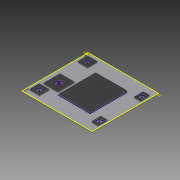
# Autodesk Inventor part: Back_part
Saved by Autodesk Inventor 2015 SP2 (Build 190223200, 223)
## iProperties
Created: 2016-11-11
Part Number: Back_part
Material: Generic
Document SubType Name: Modeling
Designer: Yann Cesbron
Density: 1 g/cm^3
Appearance: Default
Mass: 3708.65 g
Surface Area: 8125 cm^2
Volume: 3708.65 cm^3
Material: Perspex Black 9961 -10 mm
Author: Yann Cesbron
Autodesk Inventor part; units mm, degrees
ref_plane "YZ Plane" through (0, 0, 0) normal (1, 0, 0) x (0, 1, 0)
ref_plane "XZ Plane" through (0, 0, 0) normal (0, 1, 0) x (-1, 0, 0)
ref_plane "XY Plane" through (0, 0, 0) normal (0, 0, 1) x (1, 0, 0)
ref_plane "Work Plane1" through (0, 0, 0) normal (0, 0, 1) x (1, 0, 0)
sketch "Sketch1" plane through (0, 0, 0) normal (0, 0, 1) x (1, 0, 0)
  point P0 (0, 0)
ref_plane "Work Plane2" through (0, 0, 0) normal (0, 0, 1) x (1, 0, 0)
sketch "Sketch2" plane through (0, 0, 0) normal (0, 0, 1) x (1, 0, 0)
  line L0 (0, 10) -> (620, 10)
  line L1 (620, 10) -> (620, -575)
  line L2 (620, -575) -> (0, -575)
  line L3 (0, -575) -> (0, 10)
  point P0 (0, 0)
  dimension "d0" = 620
  dimension "d1" = 585
  dimension "d2" = 620
  dimension "d254" = 10
  constraints: 8 end point, 2 parallel, 1 horizontal, 1 perpendicular
  measures "d0" distance of L1.end L2.end
  measures "d1" distance between parallel lines of L0 L2
  measures "d2" distance from line of point (0, 0) L1
  measures "d254" distance from line of point (0, 0) L0
extrude "Extrusion1" add sketch "Sketch2" along normal blind 10
sketch "Excitation_port" plane through (0, 0, 10) normal (0, 0, 1) x (1, 0, 0)
  circle A0 centre (110, -357) radius 13
  line L0 (0, 10) -> (0, -575) projected
  line L1 (0, -575) -> (620, -575) projected
  circle A1 centre (110, -357) radius 30
  point P0 (0, 0)
  dimension "d6" = 26
  dimension "d7" = 110
  dimension "d8" = 218
  dimension "d9" = 60
  constraints: 2 centre point, 1 concentric
  measures "d6" diameter of A0
  measures "d7" distance from line of L0 A0.centre
  measures "d8" distance from line of L1 A0.centre
  measures "d9" diameter of A1
sketch "Air_duct_shapes_back" plane through (0, 0, 10) normal (0, 0, 1) x (1, 0, 0)
  circle A0 centre (75, -70) radius 23.5
  line L0 (0, 10) -> (0, -575) projected
  line L1 (620, 10) -> (0, 10) projected
  circle A1 centre (580, -470) radius 23.5
  circle A2 centre (580, -95) radius 23.5
  circle A3 centre (75, -495) radius 23.5
  line L2 (0, -575) -> (620, -575) projected
  line L3 (620, -575) -> (620, 10) projected
  point P0 (0, 0)
  dimension "d10" = 47
  dimension "d11" = 75
  dimension "d12" = 80
  dimension "d13" = 47
  dimension "d14" = 47
  dimension "d15" = 47
  dimension "d16" = 80
  dimension "d17" = 75
  dimension "d18" = 105
  dimension "d19" = 105
  dimension "d20" = 40
  dimension "d21" = 40
  constraints: 4 centre point
  measures "d10" diameter of A0
  measures "d11" distance from line of L0 A0.centre
  measures "d12" distance from line of L1 A0.centre
  measures "d13" diameter of A1
  measures "d14" diameter of A2
  measures "d15" diameter of A3
  measures "d16" distance from line of L2 A3.centre
  measures "d17" distance from line of L0 A3.centre
  measures "d18" distance from line of L2 A1.centre
  measures "d19" distance from line of L1 A2.centre
  measures "d20" distance from line of L3 A2.centre
  measures "d21" distance from line of L3 A1.centre
sketch "Flanges_back" plane through (0, 0, 10) normal (0, 0, 1) x (1, 0, 0)
  line L0 (620, -575) -> (620, 10) projected
  circle A0 centre (580, -95) radius 23.75
  line L1 (605, -52.5) -> (555, -52.5)
  line L2 (550, -57.5) -> (550, -132.5)
  line L3 (555, -137.5) -> (605, -137.5)
  line L4 (610, -132.5) -> (610, -57.5)
  line L5 (610, -52.5) -> (550, -137.5) construction
  line L6 (550, -52.5) -> (610, -137.5) construction
  line L7 (620, 10) -> (0, 10) projected
  circle A1 centre (580, -470) radius 23.75
  line L8 (0, -575) -> (620, -575) projected
  line L9 (555, -512.5) -> (605, -512.5)
  line L10 (610, -507.5) -> (610, -432.5)
  line L11 (605, -427.5) -> (555, -427.5)
  line L12 (550, -432.5) -> (550, -507.5)
  line L13 (550, -512.5) -> (610, -427.5) construction
  line L14 (610, -512.5) -> (550, -427.5) construction
  circle A2 centre (75, -70) radius 23.75
  line L15 (0, 10) -> (0, -575) projected
  line L16 (35, -115) -> (115, -115)
  line L17 (120, -110) -> (120, -30)
  line L18 (115, -25) -> (35, -25)
  line L19 (30, -30) -> (30, -110)
  line L20 (30, -115) -> (120, -25) construction
  line L21 (120, -115) -> (30, -25) construction
  circle A3 centre (75, -495) radius 23.75
  line L22 (35, -540) -> (115, -540)
  line L23 (120, -535) -> (120, -455)
  line L24 (115, -450) -> (35, -450)
  line L25 (30, -455) -> (30, -535)
  line L26 (30, -540) -> (120, -450) construction
  line L27 (120, -540) -> (30, -450) construction
  circle A4 centre (110, -357) radius 30
  line L28 (50, -432) -> (170, -432)
  line L29 (175, -427) -> (175, -287)
  line L30 (170, -282) -> (50, -282)
  line L31 (45, -287) -> (45, -427)
  line L32 (45, -432) -> (175, -282) construction
  line L33 (175, -432) -> (45, -282) construction
  circle A5 centre (602.5, -60) radius 2.25
  circle A6 centre (557.5, -60) radius 2.25
  circle A7 centre (557.5, -130) radius 2.25
  circle A8 centre (602.5, -130) radius 2.25
  circle A9 centre (602.5, -505) radius 2.25
  circle A10 centre (602.5, -435) radius 2.25
  circle A11 centre (557.5, -435) radius 2.25
  circle A12 centre (557.5, -505) radius 2.25
  circle A13 centre (75, -32.5) radius 2.25
  circle A14 centre (112.5, -70) radius 2.25
  circle A15 centre (75, -107.5) radius 2.25
  circle A16 centre (37.5, -70) radius 2.25
  circle A17 centre (112.5, -495) radius 2.25
  circle A18 centre (75, -532.5) radius 2.25
  circle A19 centre (75, -457.5) radius 2.25
  circle A20 centre (37.5, -495) radius 2.25
  circle A21 centre (167.5, -317) radius 2.25
  circle A22 centre (167.5, -397) radius 2.25
  circle A23 centre (110, -424.5) radius 2.25
  circle A24 centre (110, -289.5) radius 2.25
  circle A25 centre (52.5, -317) radius 2.25
  circle A26 centre (52.5, -397) radius 2.25
  arc A27 (115, -115) -> (120, -110) centre (115, -110) ccw
  arc A28 (120, -30) -> (115, -25) centre (115, -30) ccw
  arc A29 (35, -25) -> (30, -30) centre (35, -30) ccw
  arc A30 (30, -110) -> (35, -115) centre (35, -110) ccw
  arc A31 (115, -540) -> (120, -535) centre (115, -535) ccw
  arc A32 (120, -455) -> (115, -450) centre (115, -455) ccw
  arc A33 (35, -450) -> (30, -455) centre (35, -455) ccw
  arc A34 (30, -535) -> (35, -540) centre (35, -535) ccw
  arc A35 (175, -287) -> (170, -282) centre (170, -287) ccw
  arc A36 (50, -282) -> (45, -287) centre (50, -287) ccw
  arc A37 (45, -427) -> (50, -432) centre (50, -427) ccw
  arc A38 (170, -432) -> (175, -427) centre (170, -427) ccw
  arc A39 (550, -507.5) -> (555, -512.5) centre (555, -507.5) ccw
  arc A40 (605, -512.5) -> (610, -507.5) centre (605, -507.5) ccw
  arc A41 (610, -432.5) -> (605, -427.5) centre (605, -432.5) ccw
  arc A42 (555, -427.5) -> (550, -432.5) centre (555, -432.5) ccw
  arc A43 (555, -52.5) -> (550, -57.5) centre (555, -57.5) ccw
  arc A44 (610, -57.5) -> (605, -52.5) centre (605, -57.5) ccw
  arc A45 (605, -137.5) -> (610, -132.5) centre (605, -132.5) ccw
  arc A46 (550, -132.5) -> (555, -137.5) centre (555, -132.5) ccw
  point P0 (0, 0)
  point P1 (580, -95)
  point P2 (580, -470)
  point P3 (75, -495)
  point P4 (110, -357)
  dimension "d69" = 47.5
  dimension "d70" = 105
  dimension "d71" = 60
  dimension "d72" = 85
  dimension "d75" = 47.5
  dimension "d76" = 40
  dimension "d77" = 105
  dimension "d78" = 60
  dimension "d79" = 85
  dimension "d80" = 40
  dimension "d81" = 47.5
  dimension "d82" = 80
  dimension "d83" = 75
  dimension "d84" = 90
  dimension "d86" = 47.5
  dimension "d87" = 80
  dimension "d88" = 75
  dimension "d91" = 60
  dimension "d92" = 130
  dimension "d93" = 150
  dimension "d94" = 110
  dimension "d95" = 218
  dimension "d109" = 4.5
  dimension "d110" = 7.5
  dimension "d111" = 7.5
  dimension "d112" = 4.5
  dimension "d113" = 7.5
  dimension "d114" = 7.5
  dimension "d115" = 4.5
  dimension "d116" = 7.5
  dimension "d117" = 7.5
  dimension "d118" = 4.5
  dimension "d119" = 7.5
  dimension "d120" = 7.5
  dimension "d135" = 4.5
  dimension "d136" = 4.5
  dimension "d137" = 4.5
  dimension "d138" = 4.5
  dimension "d139" = 7.5
  dimension "d140" = 7.5
  dimension "d141" = 7.5
  dimension "d142" = 7.5
  dimension "d143" = 7.5
  dimension "d144" = 7.5
  dimension "d145" = 7.5
  dimension "d146" = 7.5
  dimension "d170" = 4.5
  dimension "d171" = 4.5
  dimension "d172" = 4.5
  dimension "d173" = 4.5
  dimension "d174" = 7.5
  dimension "d175" = 7.5
  dimension "d176" = 7.5
  dimension "d177" = 7.5
  dimension "d178" = 45
  dimension "d179" = 45
  dimension "d180" = 45
  dimension "d181" = 45
  dimension "d194" = 4.5
  dimension "d195" = 4.5
  dimension "d196" = 4.5
  dimension "d197" = 4.5
  dimension "d198" = 7.5
  dimension "d199" = 7.5
  constraints: 60 end point, 47 centre point, 40 point on circle, 40 point on line, 40 tangent, 16 midpoint, 15 equal radius, 10 parallel, 7 perpendicular, 5 coincident, 5 horizontal
  measures "d69" diameter of A0
  measures "d70" distance from line of L7 A0.centre
  measures "d71" distance of L5.end L6.end
  measures "d72" distance between parallel lines of L3 L1
  measures "d75" diameter of A1
  measures "d76" distance from line of L0 A1.centre
  measures "d77" distance from line of L8 A1.centre
  measures "d78" distance of L14.end L13.end
  measures "d79" distance of L13.end L14.start
  measures "d80" distance from line of L0 point (580, -95)
  measures "d81" diameter of A2
  measures "d82" distance from line of L7 A2.centre
  measures "d83" distance from line of L15 A2.centre
  measures "d84" distance of L21.end L20.end
  measures "d86" diameter of A3
  measures "d87" distance from line of L8 A3.centre
  measures "d88" distance from line of L15 A3.centre
  measures "d91" diameter of A4
  measures "d92" distance of L33.end L32.end
  measures "d93" distance of L32.end L33.start
  measures "d94" distance from line of L15 A4.centre
  measures "d95" distance from line of L8 A4.centre
  measures "d109" diameter of A5
  measures "d110" distance from line of L4 A5.centre
  measures "d111" distance from line of L1 A5.centre
  measures "d112" diameter of A6
  measures "d113" distance from line of L2 A6.centre
  measures "d114" distance from line of L1 A6.centre
  measures "d115" diameter of A7
  measures "d116" distance from line of L3 A7.centre
  measures "d117" distance from line of L2 A7.centre
  measures "d118" diameter of A8
  measures "d119" distance from line of L3 A8.centre
  measures "d120" distance from line of L4 A8.centre
  measures "d135" diameter of A9
  measures "d136" diameter of A10
  measures "d137" diameter of A11
  measures "d138" diameter of A12
  measures "d139" distance from line of A9.centre L9
  measures "d140" distance from line of L10 A9.centre
  measures "d141" distance from line of L10 A10.centre
  measures "d142" distance from line of L11 A10.centre
  measures "d143" distance from line of L12 A11.centre
  measures "d144" distance from line of L11 A11.centre
  measures "d145" distance from line of L9 A12.centre
  measures "d146" distance from line of L12 A12.centre
  measures "d170" diameter of A13
  measures "d171" diameter of A14
  measures "d172" diameter of A15
  measures "d173" diameter of A16
  measures "d174" distance from line of L17 A14.centre
  measures "d175" distance from line of L16 A15.centre
  measures "d176" distance from line of L18 A13.centre
  measures "d177" distance from line of L19 A16.centre
  measures "d178" distance from line of A14.centre L18
  measures "d179" distance from line of L17 A15.centre
  measures "d180" distance from line of L16 A16.centre
  measures "d181" distance from line of L19 A13.centre
  measures "d194" diameter of A17
  measures "d195" diameter of A18
  measures "d196" diameter of A19
  measures "d197" diameter of A20
  measures "d198" distance from line of L23 A17.centre
  measures "d199" distance from line of L22 A18.centre
sketch "Cut_out_back" plane through (0, 0, 10) normal (0, 0, 1) x (1, 0, 0)
  line L0 (620, 10) -> (0, 10) projected
  line L1 (0, 10) -> (0, -575) projected
  line L2 (557.5, -67.5) -> (602.5, -67.5)
  line L3 (607.5, -72.5) -> (607.5, -117.5)
  line L4 (602.5, -122.5) -> (557.5, -122.5)
  line L5 (552.5, -117.5) -> (552.5, -72.5)
  line L6 (552.5, -67.5) -> (607.5, -122.5) construction
  line L7 (607.5, -67.5) -> (552.5, -122.5) construction
  line L8 (557.5, -442.5) -> (602.5, -442.5)
  line L9 (607.5, -447.5) -> (607.5, -492.5)
  line L10 (602.5, -497.5) -> (557.5, -497.5)
  line L11 (552.5, -492.5) -> (552.5, -447.5)
  line L12 (552.5, -442.5) -> (607.5, -497.5) construction
  line L13 (607.5, -442.5) -> (552.5, -497.5) construction
  line L14 (0, -575) -> (620, -575) projected
  line L15 (620, -575) -> (620, 10) projected
  arc A0 (552.5, -117.5) -> (557.5, -122.5) centre (557.5, -117.5) ccw
  arc A1 (557.5, -67.5) -> (552.5, -72.5) centre (557.5, -72.5) ccw
  arc A2 (607.5, -72.5) -> (602.5, -67.5) centre (602.5, -72.5) ccw
  arc A3 (602.5, -122.5) -> (607.5, -117.5) centre (602.5, -117.5) ccw
  arc A4 (557.5, -442.5) -> (552.5, -447.5) centre (557.5, -447.5) ccw
  arc A5 (607.5, -447.5) -> (602.5, -442.5) centre (602.5, -447.5) ccw
  arc A6 (602.5, -497.5) -> (607.5, -492.5) centre (602.5, -492.5) ccw
  arc A7 (552.5, -492.5) -> (557.5, -497.5) centre (557.5, -492.5) ccw
  line L16 (65, -417) -> (155, -417)
  line L17 (160, -412) -> (160, -302)
  line L18 (155, -297) -> (65, -297)
  line L19 (60, -302) -> (60, -412)
  line L20 (60, -417) -> (160, -297) construction
  line L21 (160, -417) -> (60, -297) construction
  arc A8 (65, -297) -> (60, -302) centre (65, -302) ccw
  arc A9 (160, -302) -> (155, -297) centre (155, -302) ccw
  arc A10 (155, -417) -> (160, -412) centre (155, -412) ccw
  arc A11 (60, -412) -> (65, -417) centre (65, -412) ccw
  line L22 (100, -40) -> (50, -40)
  line L23 (45, -45) -> (45, -95)
  line L24 (50, -100) -> (100, -100)
  line L25 (105, -95) -> (105, -45)
  line L26 (105, -40) -> (45, -100) construction
  line L27 (45, -40) -> (105, -100) construction
  arc A12 (100, -100) -> (105, -95) centre (100, -95) ccw
  arc A13 (105, -45) -> (100, -40) centre (100, -45) ccw
  arc A14 (50, -40) -> (45, -45) centre (50, -45) ccw
  arc A15 (45, -95) -> (50, -100) centre (50, -95) ccw
  line L28 (100, -465) -> (50, -465)
  line L29 (45, -470) -> (45, -520)
  line L30 (50, -525) -> (100, -525)
  line L31 (105, -520) -> (105, -470)
  line L32 (105, -465) -> (45, -525) construction
  line L33 (45, -465) -> (105, -525) construction
  arc A16 (100, -525) -> (105, -520) centre (100, -520) ccw
  arc A17 (105, -470) -> (100, -465) centre (100, -470) ccw
  arc A18 (50, -465) -> (45, -470) centre (50, -470) ccw
  arc A19 (45, -520) -> (50, -525) centre (50, -520) ccw
  circle A20 centre (602.5, -130) radius 1.65
  circle A21 centre (602.5, -60) radius 1.65
  circle A22 centre (557.5, -60) radius 1.65
  circle A23 centre (557.5, -130) radius 1.65
  circle A24 centre (602.5, -505) radius 1.65
  circle A25 centre (557.5, -505) radius 1.65
  circle A26 centre (557.5, -435) radius 1.65
  circle A27 centre (602.5, -435) radius 1.65
  circle A28 centre (112.5, -70) radius 1.65
  circle A29 centre (75, -32.5) radius 1.65
  circle A30 centre (37.5, -70) radius 1.65
  circle A31 centre (75, -107.5) radius 1.65
  circle A32 centre (112.5, -495) radius 1.65
  circle A33 centre (37.5, -495) radius 1.65
  circle A34 centre (75, -532.5) radius 1.65
  circle A35 centre (75, -457.5) radius 1.65
  circle A36 centre (167.5, -317) radius 1.65
  circle A37 centre (167.5, -397) radius 1.65
  circle A38 centre (110, -424.5) radius 1.65
  circle A39 centre (52.5, -397) radius 1.65
  circle A40 centre (52.5, -317) radius 1.65
  circle A41 centre (110, -289.5) radius 1.65
  line L34 (0, 10) -> (20, 10)
  line L35 (20, 10) -> (20, -35)
  line L36 (20, -35) -> (0, -35)
  line L37 (0, -35) -> (0, 10)
  line L38 (0, -575) -> (20, -575)
  line L39 (20, -575) -> (20, -530)
  line L40 (20, -530) -> (0, -530)
  line L41 (0, -530) -> (0, -575)
  circle A42 centre (35, 5) radius 2.25
  circle A43 centre (170, 5) radius 2.25
  circle A44 centre (305, 5) radius 2.25
  circle A45 centre (440, 5) radius 2.25
  circle A46 centre (575, 5) radius 2.25
  circle A47 centre (35, -570) radius 2.25
  circle A48 centre (170, -570) radius 2.25
  circle A49 centre (305, -570) radius 2.25
  circle A50 centre (440, -570) radius 2.25
  circle A51 centre (575, -570) radius 2.25
  circle A52 centre (615, -30) radius 2.25
  circle A53 centre (615, -195) radius 2.25
  circle A54 centre (615, -370) radius 2.25
  circle A55 centre (615, -535) radius 2.25
  line L42 (220, -432.5) -> (450, -432.5)
  line L43 (460, -422.5) -> (460, -142.5)
  line L44 (450, -132.5) -> (220, -132.5)
  line L45 (210, -142.5) -> (210, -422.5)
  line L46 (210, -432.5) -> (460, -132.5) construction
  line L47 (460, -432.5) -> (210, -132.5) construction
  arc A56 (450, -432.5) -> (460, -422.5) centre (450, -422.5) ccw
  arc A57 (460, -142.5) -> (450, -132.5) centre (450, -142.5) ccw
  arc A58 (220, -132.5) -> (210, -142.5) centre (220, -142.5) ccw
  arc A59 (210, -422.5) -> (220, -432.5) centre (220, -422.5) ccw
  point P0 (0, 0)
  point P1 (580, -95)
  point P2 (580, -470)
  point P3 (110, -357)
  point P4 (75, -70)
  point P5 (75, -495)
  point P6 (335, -282.5)
  point P7 (467.5, -147.5)
  point P8 (467.5, -417.5)
  point P9 (445, -125)
  point P10 (445, -440)
  point P11 (225, -440)
  point P12 (202.5, -417.5)
  point P13 (202.5, -147.5)
  point P14 (225, -125)
  point P15 (335, -125)
  point P16 (467.5, -282.5)
  point P17 (335, -440)
  point P18 (202.5, -282.5)
  dimension "d26" = 55
  dimension "d31" = 105
  dimension "d32" = 40
  dimension "d33" = 105
  dimension "d34" = 40
  dimension "d36" = 55
  dimension "d37" = 5
  dimension "d38" = 5
  dimension "d41" = 100
  dimension "d45" = 110
  dimension "d46" = 218
  dimension "d47" = 120
  dimension "d48" = 5
  dimension "d49" = 60
  dimension "d52" = 5
  dimension "d53" = 60
  dimension "d54" = 5
  dimension "d57" = 80
  dimension "d58" = 75
  dimension "d59" = 80
  dimension "d60" = 75
  dimension "d97" = 3.3
  dimension "d98" = 7.5
  dimension "d99" = 5
  dimension "d100" = 3.3
  dimension "d101" = 3.3
  dimension "d102" = 3.3
  dimension "d105" = 45
  dimension "d108" = 7.5
  dimension "d121" = 3.3
  dimension "d122" = 3.3
  dimension "d123" = 3.3
  dimension "d124" = 3.3
  dimension "d125" = 7.5
  dimension "d126" = 7.5
  dimension "d127" = 7.5
  dimension "d130" = 5
  dimension "d131" = 45
  dimension "d133" = 45
  dimension "d147" = 7.5
  dimension "d149" = 45
  dimension "d151" = 5
  dimension "d152" = 7.5
  dimension "d153" = 5
  dimension "d156" = 7.5
  dimension "d157" = 3.3
  dimension "d158" = 3.3
  dimension "d159" = 3.3
  dimension "d160" = 3.3
  dimension "d161" = 7.5
  dimension "d162" = 7.5
  dimension "d163" = 7.5
  dimension "d164" = 7.5
  dimension "d166" = 30
  dimension "d167" = 30
  dimension "d168" = 30
  dimension "d169" = 30
  dimension "d182" = 3.3
  dimension "d183" = 3.3
  dimension "d184" = 3.3
  dimension "d185" = 3.3
  dimension "d186" = 7.5
  dimension "d187" = 7.5
  dimension "d188" = 7.5
  constraints: 88 end point, 60 centre point, 48 point on circle, 48 point on line, 48 tangent, 18 equal radius, 16 parallel, 12 midpoint, 12 perpendicular, 8 horizontal
  measures "d26" distance of L6.end L7.end
  measures "d31" distance from line of L14 point (580, -470)
  measures "d32" distance from line of L15 point (580, -470)
  measures "d33" distance from line of L0 point (580, -95)
  measures "d34" distance from line of L15 point (580, -95)
  measures "d36" distance between parallel lines of L11 L9
  measures "d37" radius of A0
  measures "d38" radius of A4
  measures "d41" distance of L21.end L20.end
  measures "d45" distance from line of L1 point (110, -357)
  measures "d46" distance from line of L14 point (110, -357)
  measures "d47" distance between parallel lines of L16 L18
  measures "d48" radius of A8
  measures "d49" distance of L27.end L26.end
  measures "d52" radius of A12
  measures "d53" distance of L33.end L32.end
  measures "d54" radius of A16
  measures "d57" distance from line of L14 point (75, -495)
  measures "d58" distance from line of L1 point (75, -495)
  measures "d59" distance from line of L0 point (75, -70)
  measures "d60" distance from line of L1 point (75, -70)
  measures "d97" diameter of A20
  measures "d98" distance from line of L4 A20.centre
  measures "d99" distance from line of L3 A20.centre
  measures "d100" diameter of A21
  measures "d101" diameter of A22
  measures "d102" diameter of A23
  measures "d105" distance of A23.centre A20.centre
  measures "d108" distance from line of L2 A22.centre
  measures "d121" diameter of A24
  measures "d122" diameter of A25
  measures "d123" diameter of A26
  measures "d124" diameter of A27
  measures "d125" distance from line of A24.centre L10
  measures "d126" distance from line of L8 A27.centre
  measures "d127" distance from line of L8 A26.centre
  measures "d130" distance from line of A24.centre L9
  measures "d131" distance of A25.centre A24.centre
  measures "d133" distance of A26.centre A27.centre
  measures "d147" distance from line of L4 A23.centre
  measures "d149" distance of A22.centre A21.centre
  measures "d151" distance from line of L3 A21.centre
  measures "d152" distance from line of L10 A25.centre
  measures "d153" distance from line of L9 A27.centre
  measures "d156" distance from line of L2 A21.centre
  measures "d157" diameter of A28
  measures "d158" diameter of A29
  measures "d159" diameter of A30
  measures "d160" diameter of A31
  measures "d161" distance from line of L25 A28.centre
  measures "d162" distance from line of L23 A30.centre
  measures "d163" distance from line of L24 A31.centre
  measures "d164" distance from line of L22 A29.centre
  measures "d166" distance from line of L23 A31.centre
  measures "d167" distance from line of A28.centre L24
  measures "d168" distance from line of L25 A29.centre
  measures "d169" distance from line of A30.centre L22
  measures "d182" diameter of A32
  measures "d183" diameter of A33
  measures "d184" diameter of A34
  measures "d185" diameter of A35
  measures "d186" distance from line of L31 A32.centre
  measures "d187" distance from line of L30 A34.centre
  measures "d188" distance from line of L29 A33.centre
extrude "Extrusion2" cut sketch "Cut_out_back" against normal blind 10 contours L15 L14 L39 L40 L1 L36 L35 L0 | A59 L45 A58 L44 A57 L43 A56 L42 keep common part
sketch "Bracket_holes_back" plane through (0, 0, 10) normal (0, 0, 1) x (1, 0, 0)
  line L0 (0, -35) -> (0, -530) projected
  line L1 (620, 10) -> (20, 10) projected
  point P0 (0, 0)
  point P1 (7.5, -270)
  dimension "d301" = 7.5
  dimension "d302" = 280
  measures "d301" distance from line of L0 point (7.5, -270)
  measures "d302" distance from line of point (7.5, -270) L1
hole "Bracket_holes_back_1" at (7.5, -270, 10) direction (0, 0, -1) diameter 3.3 end through all
extrude "Extrusion4" cut sketch "Cut_out_back" against normal blind 10 contours A59 L45 A58 L44 A57 L43 A56 L42
extrude "Extrusion6" add sketch "Flanges_back" along normal blind 10 separate body contours A44 L4 A45 L3 A46 L2 A43 L1
extrude "Extrusion7" add sketch "Flanges_back" along normal blind 10 separate body contours A39 L12 A42 L11 A41 L10 A40 L9
extrude "Extrusion8" add sketch "Flanges_back" along normal blind 10 separate body contours A37 L31 A36 L30 A35 L29 A38 L28
extrude "Extrusion9" add sketch "Flanges_back" along normal blind 10 separate body contours A34 L25 A33 L24 A32 L23 A31 L22
extrude "Extrusion10" add sketch "Flanges_back" along normal blind 10 separate body contours A30 L19 A29 L18 A28 L17 A27 L16
hole "Hole2" at (467.5, -147.5, 10) at (467.5, -417.5, 10) at (445, -125, 10) at (445, -440, 10) at (225, -440, 10) at (202.5, -417.5, 10) at (202.5, -147.5, 10) at (225, -125, 10) at (335, -125, 10) at (467.5, -282.5, 10) at (335, -440, 10) at (202.5, -282.5, 10) direction (0, 0, -1) diameter 3.3 end through all bodies 1
sketch "Opening_cover_back" plane through (0, 0, 10) normal (0, 0, 1) x (1, 0, 0)
  line L0 (465, -117.5) -> (205, -117.5)
  line L1 (195, -127.5) -> (195, -437.5)
  line L2 (205, -447.5) -> (465, -447.5)
  line L3 (475, -437.5) -> (475, -127.5)
  line L4 (0, -35) -> (0, -530) projected
  line L5 (620, 10) -> (20, 10) projected
  arc A0 (475, -127.5) -> (465, -117.5) centre (465, -127.5) ccw
  arc A1 (465, -447.5) -> (475, -437.5) centre (465, -437.5) ccw
  arc A2 (195, -437.5) -> (205, -447.5) centre (205, -437.5) ccw
  arc A3 (205, -117.5) -> (195, -127.5) centre (205, -127.5) ccw
  line L6 (450, -432.5) -> (220, -432.5) projected
  line L7 (450, -132.5) -> (220, -132.5) projected
  point P0 (0, 0)
  point P1 (195, -447.5)
  point P2 (195, -117.5)
  point P3 (475, -447.5)
  point P4 (467.5, -147.5)
  point P5 (467.5, -282.5)
  point P6 (467.5, -417.5)
  point P7 (445, -440)
  point P8 (445, -125)
  point P9 (335, -125)
  point P10 (335, -440)
  point P11 (225, -125)
  point P12 (202.5, -147.5)
  point P13 (202.5, -282.5)
  point P14 (202.5, -417.5)
  point P15 (225, -440)
  dimension "d341" = 280
  dimension "d342" = 330
  dimension "d343" = 195
  dimension "d344" = 127.5
  dimension "d345" = 10
  dimension "d346" = 7.5
  dimension "d347" = 7.5
  dimension "d348" = 7.5
  dimension "d349" = 30
  dimension "d350" = 30
  dimension "d351" = 30
  dimension "d352" = 30
  dimension "d356" = 7.5
  dimension "d357" = 140
  dimension "d358" = 140
  dimension "d359" = 7.5
  dimension "d360" = 7.5
  dimension "d361" = 7.5
  dimension "d362" = 165
  dimension "d363" = 165
  dimension "d364" = 7.5
  dimension "d366" = 7.5
  dimension "d367" = 7.5
  dimension "d368" = 7.5
  dimension "d369" = 30
  dimension "d370" = 30
  dimension "d371" = 30
  dimension "d372" = 30
  dimension "d392" = 7.5
  constraints: 8 end point, 8 point on circle, 8 tangent, 6 point on line, 4 centre point, 3 equal radius, 2 parallel, 1 horizontal, 1 perpendicular
  measures "d341" distance of point (475, -447.5) point (195, -447.5)
  measures "d342" distance of point (195, -447.5) point (195, -117.5)
  measures "d343" distance between parallel lines of L4 L1
  measures "d344" distance between parallel lines of L5 L0
  measures "d345" radius of A0
  measures "d346" distance from line of L3 point (467.5, -417.5)
  measures "d347" distance from line of L3 point (467.5, -282.5)
  measures "d348" distance from line of L3 point (467.5, -147.5)
  measures "d349" distance from line of L0 point (467.5, -147.5)
  measures "d350" distance from line of L2 point (467.5, -417.5)
  measures "d351" distance from line of L3 point (445, -440)
  measures "d352" distance from line of L3 point (445, -125)
  measures "d356" distance from line of L2 point (335, -440)
  measures "d357" distance from line of L3 point (335, -440)
  measures "d358" distance from line of L3 point (335, -125)
  measures "d359" distance from line of L0 point (445, -125)
  measures "d360" distance from line of L0 point (335, -125)
  measures "d361" distance from line of L2 point (445, -440)
  measures "d362" distance from line of L0 point (467.5, -282.5)
  measures "d363" distance from line of L0 point (202.5, -282.5)
  measures "d364" distance from line of L2 point (225, -440)
  measures "d366" distance from line of L1 point (202.5, -147.5)
  measures "d367" distance from line of L1 point (202.5, -282.5)
  measures "d368" distance from line of L1 point (202.5, -417.5)
  measures "d369" distance from line of L2 point (202.5, -417.5)
  measures "d370" distance from line of L0 point (202.5, -147.5)
  measures "d371" distance from line of L1 point (225, -125)
  measures "d372" distance from line of L1 point (225, -440)
  measures "d392" distance from line of L0 point (225, -125)
extrude "Extrusion5" add sketch "Opening_cover_back" along normal blind 10 separate body
hole "Hole4" at (467.5, -417.5, 10) at (445, -440, 10) at (467.5, -282.5, 10) at (467.5, -147.5, 10) at (445, -125, 10) at (335, -125, 10) at (335, -440, 10) at (225, -125, 10) at (202.5, -147.5, 10) at (202.5, -282.5, 10) at (202.5, -417.5, 10) at (225, -440, 10) direction (0, 0, 1) diameter 4.5 end through all bodies 1 7
